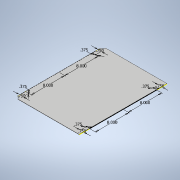
# Autodesk Inventor part: FirewallDiagonal3
Saved by Autodesk Inventor 2021 (Build 250183000, 183)
## iProperties
Created: 2020-10-29
Part Number: FirewallDiagonal3
Material: Generic
Document SubType Name: Modeling
Designer: mackeycj
Density: 1 g/cm^3
Appearance: Default
Author: mackeycj
Autodesk Inventor part; units mm, degrees
ref_plane "YZ Plane" through (0, 0, 0) normal (1, 0, 0) x (0, 1, 0)
ref_plane "XZ Plane" through (0, 0, 0) normal (0, 1, 0) x (-1, 0, 0)
ref_plane "XY Plane" through (0, 0, 0) normal (0, 0, 1) x (1, 0, 0)
sketch "Sketch1" plane through (0, 0, 0) normal (0, 1, 0) x (-1, 0, 0)
  line L0 (0, 0) -> (388.112, 0)
  line L1 (0, 0) -> (0, -266.7)
  line L2 (0, 0) -> (0, 266.7)
  line L3 (388.112, 0) -> (388.112, 266.7)
  line L4 (388.112, 0) -> (388.112, -266.7)
  line L5 (388.112, -266.7) -> (0, -266.7)
  line L6 (388.112, 266.7) -> (0, 266.7)
  line L7 (0, 266.7) -> (165.1, 266.7)
  circle A0 centre (165.1, 266.7) radius 15.875
  line L8 (165.1, 266.7) -> (294.64, 266.7)
  circle A1 centre (294.64, 266.7) radius 15.875
  circle A2 centre (388.112, 266.7) radius 15.875
  circle A3 centre (388.112, -266.7) radius 15.875
  line L9 (0, -266.7) -> (165.1, -266.7)
  line L10 (165.1, -266.7) -> (294.64, -266.7)
  circle A4 centre (165.1, -266.7) radius 15.875
  circle A5 centre (294.64, -266.7) radius 15.875
  point P0 (180.975, -266.7)
  point P1 (149.225, -266.7)
  point P2 (310.515, -266.7)
  point P3 (278.765, -266.7)
  point P4 (372.237, -266.7)
  point P5 (388.112, -250.825)
  point P6 (388.112, 250.825)
  point P7 (372.237, 266.7)
  point P8 (310.515, 266.7)
  point P9 (278.765, 266.7)
  point P10 (180.975, 266.7)
  point P11 (149.225, 266.7)
  dimension "d12" = 388.112
  dimension "d13" = 266.7
  dimension "d14" = 266.7
  dimension "d15" = 266.7
  dimension "d16" = 266.7
  dimension "d19" = 165.1
  dimension "d20" = 31.75
  dimension "d21" = 129.54
  dimension "d22" = 31.75
  dimension "d23" = 31.75
  dimension "d24" = 31.75
  dimension "d25" = 165.1
  dimension "d26" = 129.54
  dimension "d27" = 31.75
  dimension "d28" = 31.75
  constraints: 22 end point, 6 centre point, 6 coincident, 4 point on line, 4 vertical, 1 horizontal
  measures "d12" distance of L0.start L0.end
  measures "d13" distance of L0.start L1.end
  measures "d14" distance of L0.start L2.end
  measures "d15" distance of L0.end L3.end
  measures "d16" distance of L0.end L4.end
  measures "d19" distance of L2.end L7.end
  measures "d20" diameter of A0
  measures "d21" distance of L8.start L8.end
  measures "d22" diameter of A1
  measures "d23" diameter of A2
  measures "d24" diameter of A3
  measures "d25" distance of L1.end L9.end
  measures "d26" distance of L9.end L10.end
  measures "d27" diameter of A4
  measures "d28" diameter of A5
extrude "Extrusion1" add sketch "Sketch1" along normal blind 1.524 contours L2 L6 A0 A1 A2 L3 L0 | L0 L4 A3 L5 A5 A4 L1 | A4 L5 | L6 A0 | A1 L6 | L5 A5 picked at (155.2766, -262.9745) picked at (154.6704, 265.4336) picked at (284.2104, 265.4336) picked at (292.1257, -256.4991)
sketch "Sketch2" plane through (0, 0, 0) normal (0, 1, 0) x (-1, 0, 0)
  line L0 (0, 0) -> (0, 203.2)
  line L1 (0, 266.7) -> (0, -266.7) projected
  line L2 (0, 203.2) -> (19.05, 203.2)
  circle A0 centre (19.05, 203.2) radius 4.7625
  line L3 (0, 0) -> (0, -203.2)
  line L4 (0, -203.2) -> (19.05, -203.2)
  circle A1 centre (19.05, -203.2) radius 4.7625
  line L5 (388.112, -250.825) -> (388.112, 250.825) projected
  line L6 (388.112, 0) -> (388.112, 203.2)
  line L7 (388.112, 203.2) -> (369.062, 203.2)
  line L8 (388.112, 0) -> (388.112, -203.2)
  line L9 (388.112, -203.2) -> (369.062, -203.2)
  circle A2 centre (369.062, -203.2) radius 4.7625
  circle A3 centre (369.062, 203.2) radius 4.7625
  dimension "d29" = 203.2
  dimension "d30" = 19.05
  dimension "d31" = 9.525
  dimension "d32" = 203.2
  dimension "d33" = 19.05
  dimension "d34" = 9.525
  dimension "d35" = 203.2
  dimension "d36" = 19.05
  dimension "d37" = 203.2
  dimension "d38" = 19.05
  dimension "d39" = 9.525
  dimension "d40" = 9.525
  constraints: 16 end point, 4 centre point, 4 coincident, 4 perpendicular, 4 point on line, 1 midpoint
  measures "d29" distance of L0.start L0.end
  measures "d30" distance of L0.end L2.end
  measures "d31" diameter of A0
  measures "d32" distance of L0.start L3.end
  measures "d33" distance of L3.end L4.end
  measures "d34" diameter of A1
  measures "d35" distance of L6.start L6.end
  measures "d36" distance of L6.end L7.end
  measures "d37" distance of L6.start L8.end
  measures "d38" distance of L8.end L9.end
  measures "d39" diameter of A2
  measures "d40" diameter of A3
extrude "Extrusion2" [suppressed]
hole "Hole1" at (-369.062, 0, 203.2) at (-369.062, 0, -203.2) at (-19.05, 0, -203.2) at (-19.05, 0, 203.2) direction (0, 1, 0) diameter 5.1054 end through all clearance for "Flat Head Machine Screw (82)" size "#10" standard "Ansi Unified Screw Threads"
body "Solid1"
